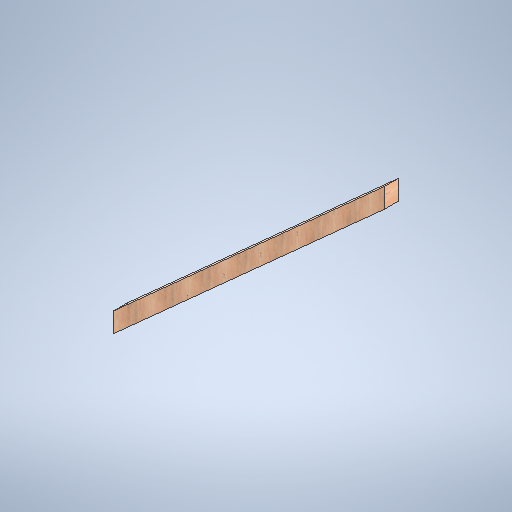
# Autodesk Inventor part: 4x4x104.303
Saved by Autodesk Inventor 2025 (Build 290162000, 162)
## iProperties
Created: 2024-08-18
Part Number: 4x4x104.303
Material: Generic
Document SubType Name: Modeling
Designer: Cupri
Density: 1 g/cm^3
Appearance: Default
Author: Cupri
Autodesk Inventor part; units mm, degrees
ref_plane "YZ Plane" through (0, 0, 0) normal (1, 0, 0) x (0, 1, 0)
ref_plane "XZ Plane" through (0, 0, 0) normal (0, 1, 0) x (-1, 0, 0)
ref_plane "XY Plane" through (0, 0, 0) normal (0, 0, 1) x (1, 0, 0)
sketch "Sketch1" plane through (0, 0, 0) normal (0, 0, 1) x (1, 0, 0)
  line L0 (-1817.394, -2192.091) -> (-1749.521, -2267.6941) construction
  line L1 (-1749.521, -2267.6941) -> (-1817.394, -2328.6274)
  line L2 (61.7703, -505.0617) -> (-1817.394, -2192.091)
  line L3 (-1749.521, -2267.6941) -> (61.7703, -641.5981)
  line L4 (61.7703, -641.5981) -> (-6.1027, -565.9951) construction
  line L5 (61.7703, -641.5981) -> (129.6433, -580.6647) construction
  line L6 (129.6433, -580.6647) -> (61.7703, -505.0617) construction
  line L7 (-1817.394, -2328.6274) -> (-1885.267, -2253.0244) construction
  line L8 (-1885.267, -2253.0244) -> (-1817.394, -2192.091) construction
  line L9 (61.7703, -505.0617) -> (61.7703, -641.5981)
  line L10 (-1817.394, -2192.091) -> (-1817.394, -2328.6274)
  dimension "d5" = 101.6
  dimension "d6" = 90
  dimension "d7" = 90
  constraints: 22 end point, 3 perpendicular, 1 point on line, 1 vertical
  measures "d5" distance of L2.end L3.start
  measures "d6" angle of L0 L2
  measures "d7" angle of L1 L0
extrude "Extrusion1" add sketch "Sketch1" along normal blind 101.6
body "Solid1"
